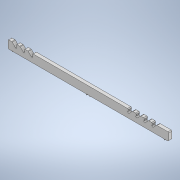
# Autodesk Inventor part: trunk
Saved by Autodesk Inventor 2020.1 (Build 241239000, 239)
## iProperties
Created: 2022-03-19
Part Number: trunk
Material: Типовые
Document SubType Name: Modeling
Designer: User
Density: 1 g/cm^3
Appearance: По умолчанию
Author: User
Autodesk Inventor part; units mm, degrees
ref_plane "YZ Plane" through (0, 0, 0) normal (1, 0, 0) x (0, 1, 0)
ref_plane "XZ Plane" through (0, 0, 0) normal (0, 1, 0) x (-1, 0, 0)
ref_plane "XY Plane" through (0, 0, 0) normal (0, 0, 1) x (1, 0, 0)
sketch "Эскиз1" plane through (0, 0, 0) normal (0, 0, 1) x (1, 0, 0)
  line L0 (0, 0) -> (-200, 0)
  line L1 (-200, 0) -> (-200, 10)
  line L2 (-200, 10) -> (0, 10)
  line L3 (0, 10) -> (0, 0)
  line L4 (-156.1916, 10) -> (-150.6349, 10) construction
  line L5 (-195, 10) -> (-188.1699, 3.1699)
  line L6 (-185, 10) -> (-178.1699, 3.1699)
  line L7 (-175, 10) -> (-168.1699, 3.1699)
  line L8 (-40, 10) -> (-34.5353, 10)
  line L9 (-30, 10) -> (-25, 10)
  line L10 (-23.8869, 10) -> (-18.8869, 10)
  line L11 (-45, 10) -> (-50, 10)
  line L12 (-200, 0) -> (-199, -1)
  line L13 (-200, 0) -> (-198.5858, 0) construction
  line L14 (-199, -1) -> (-199, 0)
  line L15 (-195, 0) -> (-195, -1)
  line L16 (-195, -1) -> (-194, 0)
  line L17 (0, 0) -> (-1, -1)
  line L18 (0, 0) -> (1.4142, 0) construction
  line L19 (-1, -1) -> (-1, 0)
  line L20 (-5, 0) -> (-5, -1)
  line L21 (-5, -1) -> (-6, 0)
  line L22 (-102, 0) -> (-102, -1)
  line L23 (-102, -1) -> (-103, 0)
  line L24 (-98, 0) -> (-98, -1)
  line L25 (-98, -1) -> (-97, 0)
  line L26 (-188.1699, 3.1699) -> (-190, 10)
  line L27 (-180, 10) -> (-178.1699, 3.1699)
  line L28 (-170, 10) -> (-168.1699, 3.1699)
  line L29 (-35, 10) -> (-41.8301, 3.1699)
  line L30 (-41.8301, 3.1699) -> (-40, 10)
  line L31 (-30, 10) -> (-31.8301, 3.1699)
  line L32 (-31.8301, 3.1699) -> (-25, 10)
  line L33 (-20, 10) -> (-21.8301, 3.1699)
  line L34 (-21.8301, 3.1699) -> (-15, 10)
  line L35 (-45, 10) -> (-51.8301, 3.1699)
  line L36 (-51.8301, 3.1699) -> (-50, 10)
  point P0 (-200, 5)
  point P1 (-100, 0)
  point P2 (-191.5849, 6.5849)
  dimension "d0" = 200
  dimension "d1" = 10
  dimension "d3" = 45
  dimension "d4" = 5
  dimension "d7" = 5
  dimension "d8" = 45
  dimension "d9" = 45
  dimension "d10" = 0
  dimension "d11" = 0
  dimension "d21" = 45
  dimension "d22" = 45
  dimension "d23" = 1
  dimension "d24" = 4
  dimension "d25" = 1
  dimension "d26" = 135
  dimension "d27" = 1
  dimension "d28" = 4
  dimension "d29" = 1
  dimension "d30" = 45
  dimension "d31" = 2
  dimension "d32" = 45
  dimension "d33" = 1
  dimension "d34" = 1
  dimension "d35" = 2
  dimension "d36" = 45
  dimension "d37" = 75
  dimension "d38" = 5
  dimension "d40" = 5
  dimension "d41" = 5
  dimension "d42" = 5
  dimension "d43" = 150
  dimension "d44" = 5
  dimension "d46" = 5
  dimension "d47" = 5
  dimension "d48" = 5
  dimension "d49" = 5
  dimension "d51" = 45
  dimension "d52" = 75
  dimension "d53" = 5
  dimension "d54" = 5
  dimension "d55" = 75
  dimension "d56" = 75
  dimension "d57" = 45
  dimension "d58" = 45
  dimension "d59" = 45
  dimension "d60" = 75
  constraints: 70 end point, 7 horizontal, 7 vertical, 3 coincident, 3 parallel, 2 equal length, 2 midpoint, 2 point on line, 26 other
  measures "d0" distance of L1.end L3.start
  measures "d1" distance of L3.start L3.end
  measures "d3" angle to the sketch x axis of L5
  measures "d4" distance of L5.start L1.end
  measures "d7" distance of L7.start L27.start
  measures "d8" angle to the sketch x axis of L6
  measures "d9" angle to the sketch x axis of L7
  measures "d10" vertical distance of L6.end L5.end
  measures "d11" vertical distance of L7.end L6.end
  measures "d21" angle of L12 L13
  measures "d22" angle of L16 L15
  measures "d23" distance of L12.end L14.end
  measures "d24" distance of L15.start L14.end
  measures "d25" distance of L15.start L15.end
  measures "d26" angle of L17 L18
  measures "d27" distance of L17.end L19.end
  measures "d28" distance of L19.end L20.start
  measures "d29" distance of L20.start L20.end
  measures "d30" angle to the sketch x axis of L21
  measures "d31" distance of point (-100, 0) L22.start
  measures "d32" angle to the sketch x axis of L23
  measures "d33" distance of L22.start L22.end
  measures "d34" distance of L24.start L24.end
  measures "d35" distance of point (-100, 0) L24.start
  measures "d36" angle to the sketch x axis of L25
  measures "d37" angle to the sketch x axis of L26
  measures "d38" distance of L26.end L5.start
  measures "d40" distance of L6.start L26.end
  measures "d41" distance of L27.start L6.start
  measures "d42" distance of L28.start L7.start
  measures "d43" distance of L8.start L26.end
  measures "d44" distance of L8.start L29.start
  measures "d46" distance of L9.start L32.end
  measures "d47" distance of L29.start L9.start
  measures "d48" distance of L33.start L32.end
  measures "d49" distance of L34.end L33.start
  measures "d51" angle to the sketch x axis of L29
  measures "d52" angle to the sketch x axis of L30
  measures "d53" distance of L35.start L8.start
  measures "d54" distance of L36.end L35.start
  measures "d55" angle to the sketch x axis of L31
  measures "d56" angle to the sketch x axis of L33
  measures "d57" angle to the sketch x axis of L34
  measures "d58" angle to the sketch x axis of L32
  measures "d59" angle to the sketch x axis of L35
  measures "d60" angle to the sketch x axis of L36
extrude "Выдавливание1" add sketch "Эскиз1" along normal blind 4 contours L17 L19 L0 | L0 L1 L2 L5 L26 L6 L27 L7 L28 L36 L35 L30 L29 L31 L32 L33 L34 L3 | L20 L21 L0 | L25 L24 L0 | L22 L23 L0 | L16 L15 L0 | L14 L12 L0
fillet "Сопряжение1" radius 1 21 edges at (-190, 10, 2) (-188.1699, 3.1699, 2) (-195, 10, 2) (-185, 10, 2) (-178.1699, 3.1699, 2) (-180, 10, 2) (-168.1699, 3.1699, 2) (-175, 10, 2) (-170, 10, 2) (-50, 10, 2) (-51.8301, 3.1699, 2) (-41.8301, 3.1699, 2) (-31.8301, 3.1699, 2) (-30, 10, 2) (-40, 10, 2) (-45, 10, 2) (-35, 10, 2) (-25, 10, 2) (-20, 10, 2) (-21.8301, 3.1699, 2) (-15, 10, 2)
fillet "Сопряжение2" radius 1 2 edges at (0, 10, 2) (-200, 10, 2)
sketch "Эскиз2" plane through (0, 0, 4) normal (0, 0, 1) x (1, 0, 0)
  line L0 (0, 0) -> (-3.077, 0)
  line L1 (-3.077, 0) -> (-3.077, -3.9049)
  line L2 (-3.077, -3.9049) -> (0, -3.9049)
  line L3 (0, -3.9049) -> (0, 0)
  line L4 (-199, 0) -> (-195, 0) projected
  line L5 (-199, 0) -> (-201.3161, 0)
  line L6 (-201.3161, 0) -> (-201.3161, -2.7777)
  line L7 (-201.3161, -2.7777) -> (-199, -2.7777)
  line L8 (-199, -2.7777) -> (-199, 0)
  constraints: 16 end point, 4 parallel, 2 horizontal, 2 perpendicular
extrude "Выдавливание2" cut sketch "Эскиз2" against normal blind 10
chamfer "Фаска1" distance 1 angle 45 2 edges at (-200, 0, 2) (0, 0, 2)
